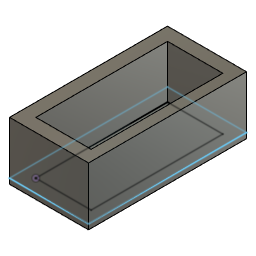
BrutalMountTest v2 (Autodesk Fusion 360 design; units mm, degrees)
Autodesk Fusion 360 part; units mm, degrees
sketch "草图1" plane through (0, 0, 0) normal (0, 1, 0) x (1, 0, 0)
  line L0 (0, 0) -> (10.5, 0)
  line L1 (10.5, 0) -> (10.5, 25)
  line L2 (10.5, 25) -> (0, 25)
  line L3 (0, 25) -> (0, 0)
  line L4 (-2.5, -2.5) -> (12.5, -2.5)
  line L5 (12.5, -2.5) -> (12.5, 27.5)
  line L6 (12.5, 27.5) -> (-2.5, 27.5)
  line L7 (-2.5, 27.5) -> (-2.5, -2.5)
  dimension "d1" = 25
  dimension "d2" = 10.5
  constraint coincident L0.start L3.end
  constraint horizontal L0
  constraint perpendicular L0 L1
  constraint perpendicular L1 L2
  constraint perpendicular L0 L3
  constraint horizontal L4
  constraint vertical L5
  constraint horizontal L6
  constraint vertical L7
  measures "d1" distance of L0.end L1.end
  measures "d2" distance of L0.start L0.end
extrude "拉伸3" add sketch "草图1" against normal blind 1 contours L0 L1 L2 L3 | L4 L5 L6 L7
extrude "拉伸4" add sketch "草图1" along normal blind 10
sketch "草图2" plane through (0, 0, 0) normal (0, 1, 0) x (1, 0, 0)
  line L0 (-2.5, -2.5) -> (-2.5, 27.5)
  line L1 (-2.5, 27.5) -> (12.5, 27.5)
  line L2 (12.5, 27.5) -> (12.5, -2.5)
  line L3 (12.5, -2.5) -> (-2.5, -2.5)
  constraint vertical L0
  constraint perpendicular L0 L1
  constraint perpendicular L1 L2
  constraint perpendicular L0 L3
extrude "拉伸1" [rolled back] along distance -2 taper angle 0
extrude "拉伸2" [rolled back] along distance 10 taper angle 0
